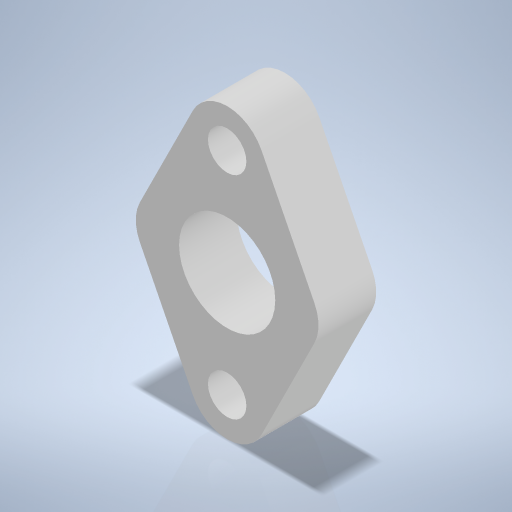
# Autodesk Inventor part: 1162
Saved by Autodesk Inventor 2024 (Build 280153000, 153)
## iProperties
Created: 2024-06-11
Part Number: 1162
Material: Generisch
Document SubType Name: Modeling
Designer: ffogue
Density: 1 g/cm^3
Appearance: Vorgabe
Author: ffogue
Autodesk Inventor part; units mm, degrees
ref_plane "YZ Plane" through (0, 0, 0) normal (1, 0, 0) x (0, 1, 0)
ref_plane "XZ Plane" through (0, 0, 0) normal (0, 1, 0) x (-1, 0, 0)
ref_plane "XY Plane" through (0, 0, 0) normal (0, 0, 1) x (1, 0, 0)
sketch "Skizze1" plane through (0, 0, 0) normal (0, 1, 0) x (-1, 0, 0)
  line L0 (0, 11) -> (0, -11) construction
  line L1 (9.5, 0) -> (-9.5, 0) construction
  arc A0 (3.5777, 12.7889) -> (-3.5777, 12.7889) centre (0, 11) ccw
  arc A1 (-3.5777, -12.7889) -> (3.5777, -12.7889) centre (0, -11) ccw
  arc A2 (9.0777, -1.7889) -> (9.0777, 1.7889) centre (5.5, 0) ccw
  arc A3 (-9.0777, 1.7889) -> (-9.0777, -1.7889) centre (-5.5, 0) ccw
  line L2 (-3.5777, 12.7889) -> (-9.0777, 1.7889)
  line L3 (3.5777, -12.7889) -> (9.0777, -1.7889)
  line L4 (9.0777, 1.7889) -> (3.5777, 12.7889)
  line L5 (-9.0777, -1.7889) -> (-3.5777, -12.7889)
  point P0 (0, 0)
  point P1 (0, 0)
  point P2 (0, -15)
  point P3 (0, 15)
  dimension "d4" = 19
  dimension "d5" = 22
  dimension "d6" = 4
  dimension "d7" = 4
  dimension "d8" = 4
  dimension "d9" = 4
  dimension "d10" = 30
  constraints: 12 end point, 12 point on circle, 8 tangent, 4 centre point, 3 coincident, 2 midpoint, 1 horizontal, 1 vertical
  measures "d4" distance of L1.end L1.start
  measures "d5" distance of L0.start L0.end
  measures "d6" radius of A0
  measures "d7" radius of A1
  measures "d8" radius of A2
  measures "d9" radius of A3
  measures "d10" distance of point (0, -15) point (0, 15)
extrude "Extrusion1" add sketch "Skizze1" along normal blind 6
sketch "Skizze2" plane through (0, 6, 0) normal (0, 1, 0) x (1, 0, 0)
  arc A0 (-3.5777, -12.7889) -> (3.5777, -12.7889) centre (0, -11) ccw projected
  arc A1 (3.5777, 12.7889) -> (-3.5777, 12.7889) centre (0, 11) ccw projected
  point P0 (0, 0)
  constraints: 2 coincident
hole "Bohrung1" at (0, 6, 11) at (0, 6, -11) direction (0, -1, 0) diameter 4 depth 6
sketch "Skizze3" plane through (0, 6, 0) normal (0, 1, 0) x (1, 0, 0)
  point P0 (0, 0)
  point P1 (0, 0)
  constraints: 1 coincident
hole "Bohrung2" at (0, 6, 0) direction (0, -1, 0) diameter 10 end through all
equation "\"d6\" = d7"
equation "\"d9\" = d8"
